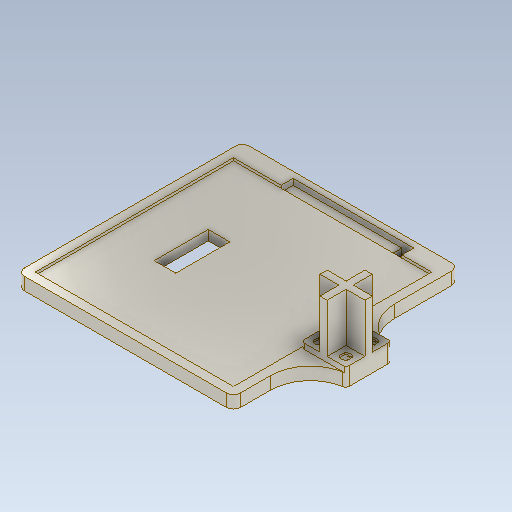
# Autodesk Inventor part: Sun1
Saved by Autodesk Inventor 2021 (Build 250183000, 183)
## iProperties
Created: 2021-04-13
Part Number: Sun1
Material: 티타늄
Document SubType Name: Modeling
Designer: Dongyoon
Density: 4.51 g/cm^3
Appearance: 티타늄
Author: Dongyoon
Autodesk Inventor part; units mm, degrees
ref_plane "YZ Plane" through (0, 0, 0) normal (1, 0, 0) x (0, 1, 0)
sketch "스케치1" plane through (0, 0, 0) normal (0, 1, 0) x (-1, 0, 0)
  line L0 (0, 0) -> (150, 0)
  line L1 (150, 0) -> (150, -140)
  line L2 (150, -140) -> (0, -140)
  line L3 (0, 0) -> (0, -140)
  dimension "d1" = 140
  dimension "d75" = 150
  constraints: 8 end point, 3 perpendicular, 1 horizontal
  measures "d1" distance between parallel lines of L2 L0
  measures "d75" distance between parallel lines of L1 L3
extrude "돌출1" add sketch "스케치1" along normal blind 7
sketch "스케치2" plane through (0, 7, 0) normal (0, 1, 0) x (1, 0, 0)
  line L0 (-145, 130) -> (-25, 130)
  line L1 (-25, 130) -> (-25, 10)
  line L2 (-25, 10) -> (-145, 10)
  line L3 (-145, 10) -> (-145, 130)
  line L4 (-150, 140) -> (-150, 0) projected
  line L5 (0, 140) -> (-150, 140) projected
  point P0 (0, 0)
  dimension "d7" = 120
  dimension "d8" = 120
  dimension "d9" = 5
  dimension "d10" = 10
  constraints: 8 end point, 2 parallel, 1 horizontal, 1 perpendicular
  measures "d7" distance of L1.end L2.end
  measures "d8" distance of L2.end L0.start
  measures "d9" distance between parallel lines of L4 L3
  measures "d10" distance between parallel lines of L5 L0
extrude "돌출2" cut sketch "스케치2" against normal blind 1.5
sketch "스케치3" plane through (0, 7, 0) normal (0, 1, 0) x (1, 0, 0)
  circle A0 centre (-5.25, 77.25) radius 2.55
  line L0 (-7.5, 78.45) -> (-7.5, 76.05)
  line L1 (-3, 76.05) -> (-3, 78.45)
  line L2 (0, 140) -> (-150, 140) projected
  line L3 (-150, 140) -> (-150, 0) projected
  circle A1 centre (-19.75, 62.75) radius 2.55
  line L4 (-22, 63.95) -> (-22, 61.55)
  line L5 (-17.5, 61.55) -> (-17.5, 63.95)
  circle A2 centre (-19.75, 77.25) radius 2.55
  line L6 (-22, 78.45) -> (-22, 76.05)
  line L7 (-17.5, 76.05) -> (-17.5, 78.45)
  circle A3 centre (-5.25, 62.75) radius 2.55
  line L8 (-7.5, 63.95) -> (-7.5, 61.55)
  line L9 (-3, 61.55) -> (-3, 63.95)
  line L10 (-150, 0) -> (0, 0) projected
  line L11 (-25, 130) -> (-25, 10) projected
  line L12 (0, 0) -> (0, 140) projected
  line L13 (-25, 72) -> (0, 72)
  line L14 (-25, 68) -> (0, 68)
  line L15 (-12.5, 72) -> (-12.5, 94.2328)
  line L16 (-12.5, 68) -> (-12.5, 31.3969)
  line L17 (-14.5, 71.4203) -> (-14.5, 94.2328)
  line L18 (-10.5, 71.4203) -> (-10.5, 94.2328)
  line L19 (-14.5, 68) -> (-14.5, 31.3969)
  line L20 (-10.5, 68) -> (-10.5, 31.3969)
  line L21 (-25, 10) -> (-145, 10) projected
  dimension "d13" = 5.1
  dimension "d14" = 4.5
  dimension "d17" = 2.25
  dimension "d18" = 5.1
  dimension "d19" = 4.5
  dimension "d20" = 2.25
  dimension "d21" = 5.1
  dimension "d22" = 4.5
  dimension "d23" = 2.25
  dimension "d24" = 5.1
  dimension "d25" = 4.5
  dimension "d26" = 2.25
  dimension "d99" = 2
  dimension "d100" = 2
  dimension "d101" = 2
  dimension "d102" = 2
  dimension "d107" = 58
  dimension "d108" = 4
  dimension "d112" = 5.25
  dimension "d113" = 5.25
  constraints: 32 end point, 16 point on circle, 8 parallel, 6 vertical, 4 centre point, 2 midpoint
  measures "d13" diameter of A0
  measures "d14" distance between parallel lines of L0 L1
  measures "d17" distance from line of A0.centre L0
  measures "d18" diameter of A1
  measures "d19" distance between parallel lines of L4 L5
  measures "d20" distance from line of A1.centre L4
  measures "d21" diameter of A2
  measures "d22" distance between parallel lines of L6 L7
  measures "d23" distance from line of A2.centre L6
  measures "d24" diameter of A3
  measures "d25" distance between parallel lines of L8 L9
  measures "d26" distance from line of A3.centre L8
  measures "d99" distance between parallel lines of L15 L17
  measures "d100" distance between parallel lines of L15 L18
  measures "d101" distance between parallel lines of L16 L19
  measures "d102" distance between parallel lines of L16 L20
  measures "d107" distance between parallel lines of L21 L14
  measures "d108" distance between parallel lines of L14 L13
  measures "d112" distance from line of L12 A0.centre
  measures "d113" distance from line of L13 A0.centre
extrude "돌출3" cut sketch "스케치3" against normal blind 1 contours L1 A0 L0 | L5 A1 L4 | L7 A2 L6 | L9 A3 L8
sketch "스케치4" plane through (0, 6, 0) normal (0, 1, 0) x (1, 0, 0)
  arc A0 (-17.5, 63.95) -> (-22, 63.95) centre (-19.75, 62.75) ccw projected
  line L0 (-19.3059, 60.239) -> (-20.1941, 65.261) construction
  line L1 (-20.1941, 60.239) -> (-19.3059, 65.261) construction
  arc A1 (-19.3059, 65.261) -> (-20.1941, 65.261) centre (-19.75, 62.75) ccw
  arc A2 (-20.1941, 60.239) -> (-19.3059, 60.239) centre (-19.75, 62.75) ccw
  line L2 (-19.3059, 61.3293) -> (-20.1941, 61.3293)
  line L3 (-20.1941, 64.1707) -> (-19.3059, 64.1707)
  line L4 (-19.3059, 61.3293) -> (-20.1941, 64.1707) construction
  line L5 (-20.1941, 61.3293) -> (-19.3059, 64.1707) construction
  line L6 (-19.3059, 65.261) -> (-19.3059, 64.1707)
  line L7 (-19.3059, 61.3293) -> (-19.3059, 60.239)
  line L8 (-20.1941, 60.239) -> (-20.1941, 61.3293)
  line L9 (-20.1941, 64.1707) -> (-20.1941, 65.261)
  arc A3 (-3, 63.95) -> (-7.5, 63.95) centre (-5.25, 62.75) ccw projected
  arc A4 (-17.5, 78.45) -> (-22, 78.45) centre (-19.75, 77.25) ccw projected
  arc A5 (-3, 78.45) -> (-7.5, 78.45) centre (-5.25, 77.25) ccw projected
  line L10 (-4.8059, 60.239) -> (-5.6941, 65.261) construction
  line L11 (-5.6941, 60.239) -> (-4.8059, 65.261) construction
  arc A6 (-4.8059, 65.261) -> (-5.6941, 65.261) centre (-5.25, 62.75) ccw
  arc A7 (-5.6941, 60.239) -> (-4.8059, 60.239) centre (-5.25, 62.75) ccw
  line L12 (-4.8059, 61.3293) -> (-5.6941, 61.3293)
  line L13 (-5.6941, 64.1707) -> (-4.8059, 64.1707)
  line L14 (-4.8059, 61.3293) -> (-5.6941, 64.1707) construction
  line L15 (-5.6941, 61.3293) -> (-4.8059, 64.1707) construction
  line L16 (-4.8059, 65.261) -> (-4.8059, 64.1707)
  line L17 (-4.8059, 61.3293) -> (-4.8059, 60.239)
  line L18 (-5.6941, 60.239) -> (-5.6941, 61.3293)
  line L19 (-5.6941, 64.1707) -> (-5.6941, 65.261)
  line L20 (-19.3059, 74.739) -> (-20.1941, 79.761) construction
  line L21 (-20.1941, 74.739) -> (-19.3059, 79.761) construction
  arc A8 (-19.3059, 79.761) -> (-20.1941, 79.761) centre (-19.75, 77.25) ccw
  arc A9 (-20.1941, 74.739) -> (-19.3059, 74.739) centre (-19.75, 77.25) ccw
  line L22 (-19.3059, 75.8293) -> (-20.1941, 75.8293)
  line L23 (-20.1941, 78.6707) -> (-19.3059, 78.6707)
  line L24 (-19.3059, 75.8293) -> (-20.1941, 78.6707) construction
  line L25 (-20.1941, 75.8293) -> (-19.3059, 78.6707) construction
  line L26 (-19.3059, 79.761) -> (-19.3059, 78.6707)
  line L27 (-19.3059, 75.8293) -> (-19.3059, 74.739)
  line L28 (-20.1941, 74.739) -> (-20.1941, 75.8293)
  line L29 (-20.1941, 78.6707) -> (-20.1941, 79.761)
  line L30 (-4.8059, 74.739) -> (-5.6941, 79.761) construction
  line L31 (-5.6941, 74.739) -> (-4.8059, 79.761) construction
  arc A10 (-4.8059, 79.761) -> (-5.6941, 79.761) centre (-5.25, 77.25) ccw
  arc A11 (-5.6941, 74.739) -> (-4.8059, 74.739) centre (-5.25, 77.25) ccw
  line L32 (-4.8059, 75.8293) -> (-5.6941, 75.8293)
  line L33 (-5.6941, 78.6707) -> (-4.8059, 78.6707)
  line L34 (-4.8059, 75.8293) -> (-5.6941, 78.6707) construction
  line L35 (-5.6941, 75.8293) -> (-4.8059, 78.6707) construction
  line L36 (-4.8059, 79.761) -> (-4.8059, 78.6707)
  line L37 (-4.8059, 75.8293) -> (-4.8059, 74.739)
  line L38 (-5.6941, 74.739) -> (-5.6941, 75.8293)
  line L39 (-5.6941, 78.6707) -> (-5.6941, 79.761)
  line L40 (-22, 61.55) -> (-22, 63.95) projected
  line L41 (-17.5, 63.95) -> (-17.5, 61.55) projected
  line L42 (-3, 63.95) -> (-3, 61.55) projected
  line L43 (-7.5, 61.55) -> (-7.5, 63.95) projected
  line L44 (-17.5, 78.45) -> (-17.5, 76.05) projected
  line L45 (-3, 78.45) -> (-3, 76.05) projected
  point P0 (0, 0)
  point P1 (-19.3059, 79.761)
  point P2 (-20.1941, 79.761)
  point P3 (-4.8059, 65.261)
  point P4 (-5.6941, 65.261)
  point P5 (-19.3059, 65.261)
  dimension "d43" = 1.8059
  dimension "d44" = 1.8059
  dimension "d45" = 2.8414
  dimension "d46" = 2.55
  dimension "d47" = 2.25
  dimension "d48" = 1.0903
  dimension "d49" = 1.1293
  dimension "d50" = 2.8414
  dimension "d51" = 1.4207
  dimension "d52" = 0.8882
  dimension "d53" = 1.8059
  dimension "d55" = 1.4207
  dimension "d56" = 1.8059
  dimension "d57" = 2.25
  dimension "d58" = 2.55
  dimension "d59" = 1.0903
  dimension "d60" = 1.4207
  dimension "d61" = 2.8414
  dimension "d62" = 0.8882
  dimension "d63" = 0.8882
  dimension "d64" = 1.0903
  dimension "d65" = 1.0903
  dimension "d66" = 1.4207
  dimension "d67" = 1.8059
  dimension "d68" = 1.8059
  dimension "d69" = 1.8059
  dimension "d70" = 2.8414
  dimension "d71" = 1.4207
  dimension "d72" = 1.8059
  dimension "d73" = 0.8882
  dimension "d74" = 0.8882
  constraints: 80 end point, 20 parallel, 18 point on circle, 10 midpoint, 8 centre point, 4 horizontal
  measures "d43" distance between parallel lines of L40 L9
  measures "d44" distance between parallel lines of L41 L6
  measures "d45" distance between parallel lines of L2 L3
  measures "d46" radius of A1
  measures "d47" distance from line of L40 A2.centre
  measures "d48" distance of L1.start L2.end
  measures "d49" distance edge to line of A2 L2
  measures "d50" distance between parallel lines of L12 L13
  measures "d51" distance from line of L13 A6.centre
  measures "d52" distance between parallel lines of L19 L16
  measures "d53" distance between parallel lines of L42 L16
  measures "d55" distance from line of L12 A7.centre
  measures "d56" distance between parallel lines of L43 L18
  measures "d57" distance from line of L43 A6.centre
  measures "d58" radius of A6
  measures "d59" distance from line of L13 L16.start
  measures "d60" distance from line of A3.centre L12
  measures "d61" distance between parallel lines of L22 L23
  measures "d62" distance between parallel lines of L26 L29
  measures "d63" distance between parallel lines of L28 L27
  measures "d64" distance of L26.start L26.end
  measures "d65" distance of L27.start L27.end
  measures "d66" distance from line of A4.centre L22
  measures "d67" distance between parallel lines of L44 L26
  measures "d68" distance between parallel lines of L44 L27
  measures "d69" distance between parallel lines of L45 L36
  measures "d70" distance between parallel lines of L32 L33
  measures "d71" distance from line of L32 A5.centre
  measures "d72" distance between parallel lines of L45 L37
  measures "d73" distance between parallel lines of L38 L37
  measures "d74" distance between parallel lines of L36 L39
extrude "돌출4" cut sketch "스케치4" against normal through all both and the other way through all
sketch "스케치6" plane through (0, 5.5, 0) normal (0, 1, 0) x (1, 0, 0)
  line L0 (-107, 60) -> (-119, 60)
  line L1 (-119, 60) -> (-119, 90)
  line L2 (-119, 90) -> (-107, 90)
  line L3 (-107, 90) -> (-107, 60)
  line L4 (-107, 60) -> (-119, 90) construction
  line L5 (-119, 60) -> (-107, 90) construction
  line L6 (-145, 130) -> (-25, 130) projected
  line L7 (-145, 10) -> (-145, 130) projected
  point P0 (0, 0)
  point P1 (-113, 75)
  dimension "d37" = 12
  dimension "d38" = 30
  dimension "d39" = 55
  dimension "d40" = 32
  constraints: 12 end point, 2 midpoint, 2 parallel, 1 horizontal, 1 perpendicular
  measures "d37" distance of L1.end L2.end
  measures "d38" distance of L2.end L0.start
  measures "d39" distance from line of L6 point (-113, 75)
  measures "d40" distance from line of L7 point (-113, 75)
extrude "돌출5" cut sketch "스케치6" against normal through all
sketch "스케치9" plane through (0, 7, 0) normal (0, 1, 0) x (1, 0, 0)
  line L0 (-25, 130) -> (-25, 10) projected
  line L1 (0, 0) -> (0, 140) projected
  line L2 (-14.5, 82.5) -> (-14.5, 72)
  line L3 (-14.5, 68) -> (-14.5, 57.5)
  line L4 (-10.5, 82.5) -> (-10.5, 72)
  line L5 (-10.5, 68) -> (-10.5, 57.5)
  line L6 (-25, 72) -> (-14.5, 72)
  line L7 (-10.5, 72) -> (0, 72)
  line L8 (-25, 68) -> (-14.5, 68)
  line L9 (-10.5, 68) -> (0, 68)
  line L10 (-25, 10) -> (-145, 10) projected
  line L11 (-145, 130) -> (-25, 130) projected
  line L12 (-14.5, 82.5) -> (-10.5, 82.5)
  line L13 (0, 72) -> (0, 68)
  line L14 (-10.5, 57.5) -> (-14.5, 57.5)
  line L15 (-25, 68) -> (-25, 72)
  line L16 (-25, 130) -> (-25, 10) projected
  point P0 (0, 68)
  point P1 (0, 72)
  dimension "d82" = 4
  dimension "d83" = 4
  dimension "d84" = 10.5
  dimension "d85" = 10.5
  dimension "d86" = 58
  dimension "d87" = 4
  dimension "d88" = 10.5
  dimension "d90" = 10.5
  dimension "d91" = 10.5
  dimension "d92" = 58
  dimension "d93" = 10.5
  dimension "d94" = 10.5
  constraints: 24 end point, 1 collinear, 1 perpendicular
  measures "d82" distance between parallel lines of L8 L6
  measures "d83" distance between parallel lines of L4 L2
  measures "d84" distance between parallel lines of L2 L0
  measures "d85" distance between parallel lines of L3 L0
  measures "d86" distance between parallel lines of L10 L8
  measures "d87" distance between parallel lines of L9 L7
  measures "d88" distance between parallel lines of L1 L5
  measures "d90" distance of L3.start L3.end
  measures "d91" distance of L5.start L5.end
  measures "d92" distance between parallel lines of L10 L9
  measures "d93" distance of L4.start L4.end
  measures "d94" distance of L2.start L2.end
extrude "돌출6" add sketch "스케치9" along normal blind 30
sketch "스케치11" plane through (-14.5, 7, -68) normal (-1, 0, 0) x (0, 0, 1)
  line L0 (0, 0) -> (0, 30) projected
  line L1 (0, 0) -> (10.5, 0)
  line L2 (10.5, 0) -> (10.5, 3)
  line L3 (10.5, 3) -> (0, 3)
  line L4 (0, 3) -> (0, 0)
  point P0 (68, -7)
  point P1 (0, 3)
  dimension "d116" = 10.5
  dimension "d117" = 3
  constraints: 8 end point, 2 parallel, 1 horizontal, 1 perpendicular
  measures "d116" distance of L2.end L3.end
  measures "d117" distance of L1.end L2.end
extrude "돌출7" add sketch "스케치11" along normal up to surface (10.5 mm away)
sketch "스케치12" plane through (-14.5, 10, -57.5) normal (0, 1, 0) x (1, 0, 0)
  arc A0 (-3, 6.45) -> (-7.5, 6.45) centre (-5.25, 5.25) ccw projected
  circle A1 centre (-5.25, 5.25) radius 2.55
  line L0 (-7.5, 4.05) -> (-7.5, 6.45) projected
  line L1 (-7.5, 6.45) -> (-7.5, 4.05)
  line L2 (-3, 6.45) -> (-3, 4.05) projected
  line L3 (-3, 4.05) -> (-3, 6.45)
  point P0 (14.5, -57.5)
  constraints: 4 end point, 1 centre point, 1 coincident, 1 collinear, 1 point on circle
extrude "돌출8" cut sketch "스케치12" against normal blind 3 contours L2 A1 L0 A0
ref_plane "작업 평면1" through (-12.5, 7, -57.5) normal (1, 0, 0) x (0, 0, -1)
mirror "미러1" about plane through (-12.5, 7, -57.5) normal (1, 0, 0) of "돌출8", "돌출7"
ref_plane "작업 평면2" through (-10.5, 37, -70) normal (0, 0, 1) x (1, 0, 0)
mirror "미러2" about plane through (-10.5, 37, -70) normal (0, 0, 1) of "돌출8", "돌출7", "미러1"
sketch "스케치13" plane through (0, 7, 0) normal (0, 1, 0) x (1, 0, 0)
  line L0 (-14.5, 57.5) -> (-25, 57.5) projected
  line L1 (-20, 35.5911) -> (-20, 0)
  line L2 (-150, 0) -> (0, 0) projected
  line L3 (-25, 57.5) -> (-25, 10) projected
  line L4 (-10.5, 57.5) -> (0, 57.5) projected
  arc A0 (0, 57.5) -> (-20, 35.5911) centre (2, 35.5911) ccw
  line L5 (0, 0) -> (0, 57.5) projected
  line L6 (0, 57.5) -> (0, 0)
  line L7 (0, 0) -> (-20, 0)
  dimension "d122" = 5
  dimension "d123" = 22
  constraints: 6 end point, 2 point on circle, 2 vertical, 1 centre point, 1 collinear, 1 point on line, 1 tangent
  measures "d122" distance between parallel lines of L3 L1
  measures "d123" radius of A0
extrude "돌출9" cut sketch "스케치13" against normal through all
mirror "미러3" about plane through (-10.5, 37, -70) normal (0, 0, 1) of "돌출9"
sketch "스케치14" plane through (0, 7, 0) normal (0, 1, 0) x (1, 0, 0)
  line L0 (-145, 130) -> (-25, 130) projected
  line L1 (-108.5, 130) -> (-41.5, 130)
  line L2 (-41.5, 130) -> (-41.5, 136.6)
  line L3 (-41.5, 136.6) -> (-108.5, 136.6)
  line L4 (-108.5, 136.6) -> (-108.5, 130)
  line L5 (-145, 10) -> (-145, 130) projected
  point P0 (0, 0)
  dimension "d126" = 67
  dimension "d127" = 6.6
  dimension "d128" = 36.5
  constraints: 8 end point, 2 parallel, 1 horizontal, 1 perpendicular, 1 point on line
  measures "d126" distance of L2.end L3.end
  measures "d127" distance of L3.end L1.start
  measures "d128" distance between parallel lines of L5 L4
extrude "돌출10" cut sketch "스케치14" against normal blind 3.3
sketch "스케치15" plane through (0, 3.7, 0) normal (0, 1, 0) x (1, 0, 0)
  line L0 (-108.5, 136.6) -> (-41.5, 136.6) projected
  line L1 (-108.5, 130) -> (-41.5, 130) projected
  line L2 (-41.5, 136.6) -> (-48.1, 136.6)
  line L3 (-48.1, 136.6) -> (-48.1, 130)
  line L4 (-48.1, 130) -> (-41.5, 130)
  line L5 (-41.5, 130) -> (-41.5, 136.6)
  point P0 (0, 0)
  dimension "d131" = 6.6
  constraints: 8 end point, 2 parallel, 1 horizontal, 1 perpendicular, 1 point on line
  measures "d131" distance between parallel lines of L5 L3
extrude "돌출11" cut sketch "스케치15" against normal through all
chamfer "모따기1" distance 5 angle 45 1 edges at (-41.5, 0, -133.3)
fillet "모깎기1" radius 2 5 edges at (0, 3.5, -57.5) (0, 3.5, -82.5) (-25, 8.5, -57.5) (-25, 8.5, -82.5) (0, 8.5, -57.5)
sketch "스케치16" plane through (0, 7, 0) normal (0, 1, 0) x (1, 0, 0)
  line L0 (-20, 35.5911) -> (-20, 0) projected
  line L1 (-150, 140) -> (-150, 0) projected
  line L2 (-20, 0) -> (-150, 0)
  line L3 (-150, 0) -> (-150, 5)
  line L4 (-150, 5) -> (-20, 5)
  line L5 (-20, 5) -> (-20, 0)
  line L6 (-25, 10) -> (-145, 10) projected
  point P0 (0, 0)
  dimension "d138" = 5
  constraints: 8 end point, 2 parallel, 1 horizontal, 1 perpendicular, 1 point on line
  measures "d138" distance between parallel lines of L6 L4
extrude "돌출12" cut sketch "스케치16" against normal through all
fillet "모깎기2" radius 4 4 edges at (-150, 3.5, -5) (-20, 3.5, -5) (-20, 3.5, -140) (-150, 3.5, -140)
sketch "스케치17" plane through (0, 6, 0) normal (0, 1, 0) x (1, 0, 0)
  arc A0 (-17.5, 63.95) -> (-22, 63.95) centre (-19.75, 62.75) ccw projected
  circle A1 centre (-19.75, 62.75) radius 2.55
  arc A2 (-22, 61.55) -> (-17.5, 61.55) centre (-19.75, 62.75) ccw projected
  line L0 (-22, 63.95) -> (-22, 61.55)
  line L1 (-17.5, 63.95) -> (-17.5, 61.55)
  line L2 (-20.1941, 61.3293) -> (-20.1941, 60.239) projected
  line L3 (-19.3059, 61.3293) -> (-20.1941, 61.3293) projected
  line L4 (-20.1941, 60.239) -> (-20.1941, 61.3293)
  line L5 (-19.3059, 60.239) -> (-19.3059, 61.3293) projected
  line L6 (-20.1941, 61.3293) -> (-19.3059, 61.3293)
  line L7 (-19.3059, 61.3293) -> (-19.3059, 60.239)
  line L8 (-20.1941, 65.261) -> (-20.1941, 64.1707) projected
  line L9 (-20.1941, 64.1707) -> (-19.3059, 64.1707) projected
  line L10 (-20.1941, 65.261) -> (-20.1941, 64.1707)
  line L11 (-20.1941, 64.1707) -> (-19.3059, 64.1707)
  line L12 (-19.3059, 64.1707) -> (-19.3059, 65.261)
  line L13 (-7.5, 61.55) -> (-7.5, 63.95) projected
  line L14 (-7.5, 63.95) -> (-7.5, 61.55)
  line L15 (-7.5, 76.05) -> (-7.5, 78.45) projected
  arc A3 (-7.5, 76.05) -> (-3, 76.05) centre (-5.25, 77.25) ccw projected
  line L16 (-7.5, 78.45) -> (-7.5, 76.05)
  arc A4 (-17.5, 78.45) -> (-22, 78.45) centre (-19.75, 77.25) ccw projected
  arc A5 (-22, 76.05) -> (-17.5, 76.05) centre (-19.75, 77.25) ccw projected
  line L17 (-22, 78.45) -> (-22, 76.05)
  circle A6 centre (-5.25, 62.75) radius 2.55
  line L18 (-7.5, 63.95) -> (-7.5, 61.55)
  line L19 (-3, 63.95) -> (-3, 61.55)
  line L20 (-5.6941, 60.239) -> (-5.6941, 61.3293)
  line L21 (-5.6941, 61.3293) -> (-4.8059, 61.3293)
  line L22 (-4.8059, 61.3293) -> (-4.8059, 60.239)
  line L23 (-5.6941, 65.261) -> (-5.6941, 64.1707)
  line L24 (-5.6941, 64.1707) -> (-4.8059, 64.1707)
  line L25 (-4.8059, 64.1707) -> (-4.8059, 65.261)
  circle A7 centre (-5.25, 77.25) radius 2.55
  line L26 (-7.5, 78.45) -> (-7.5, 76.05)
  line L27 (-3, 78.45) -> (-3, 76.05)
  line L28 (-5.6941, 74.739) -> (-5.6941, 75.8293)
  line L29 (-5.6941, 75.8293) -> (-4.8059, 75.8293)
  line L30 (-4.8059, 75.8293) -> (-4.8059, 74.739)
  line L31 (-5.6941, 79.761) -> (-5.6941, 78.6707)
  line L32 (-5.6941, 78.6707) -> (-4.8059, 78.6707)
  line L33 (-4.8059, 78.6707) -> (-4.8059, 79.761)
  circle A8 centre (-19.75, 77.25) radius 2.55
  line L34 (-22, 78.45) -> (-22, 76.05)
  line L35 (-17.5, 78.45) -> (-17.5, 76.05)
  line L36 (-20.1941, 74.739) -> (-20.1941, 75.8293)
  line L37 (-20.1941, 75.8293) -> (-19.3059, 75.8293)
  line L38 (-19.3059, 75.8293) -> (-19.3059, 74.739)
  line L39 (-20.1941, 79.761) -> (-20.1941, 78.6707)
  line L40 (-20.1941, 78.6707) -> (-19.3059, 78.6707)
  line L41 (-19.3059, 78.6707) -> (-19.3059, 79.761)
  point P0 (0, 0)
  point P1 (-3, 76.05)
  constraints: 70 end point, 15 perpendicular, 11 vertical, 9 point on circle, 4 centre point, 1 coincident
extrude "돌출13" add sketch "스케치17" along normal blind 3 contours L1 A1 L5 L3 L2 L0 A0 L8 L9 L12 | L13 A6 L23 L24 L25 L19 L22 L21 L20 | L15 A7 L31 L32 L33 L27 A3 L30 L29 L28 | L35 A5 L38 L37 L36 L17 A4 L39 L40 L41
sketch "스케치19" plane through (0, 5.5, 0) normal (0, 1, 0) x (1, 0, 0)
  line L0 (-41.5, 130) -> (-25, 130) projected
  line L1 (-25, 130) -> (-135, 130)
  line L2 (-135, 130) -> (-135, 20)
  line L3 (-135, 20) -> (-25, 20)
  line L4 (-25, 20) -> (-25, 130)
  line L5 (-145, 10) -> (-145, 130) projected
  line L6 (-135, 130) -> (-145, 130)
  line L7 (-25, 10) -> (-145, 10) projected
  line L8 (-145, 130) -> (-145, 10)
  line L9 (-145, 10) -> (-25, 10)
  line L10 (-25, 10) -> (-25, 20)
  line L11 (-20, 35.5911) -> (-20, 9) projected
  point P0 (0, 0)
  dimension "d144" = 110
  dimension "d145" = 110
  constraints: 16 end point, 4 perpendicular, 3 parallel, 1 horizontal
  measures "d144" distance of L2.end L3.end
  measures "d145" distance of L1.end L2.end
extrude "돌출14" add sketch "스케치19" along normal up to surface (1.5 mm away) contours L2 L3 L10 L7 L5 L6
sketch "스케치20" plane through (0, 5.5, 0) normal (0, 1, 0) x (1, 0, 0)
  line L0 (-107, 90) -> (-119, 90) projected
  line L1 (-109, 90) -> (-97, 90)
  line L2 (-97, 90) -> (-97, 60)
  line L3 (-97, 60) -> (-109, 60)
  line L4 (-109, 60) -> (-109, 90)
  line L5 (-135, 130) -> (-135, 20) projected
  point P0 (0, 0)
  dimension "d151" = 12
  dimension "d152" = 30
  dimension "d153" = 26
  constraints: 8 end point, 2 parallel, 1 horizontal, 1 perpendicular, 1 point on line
  measures "d151" distance of L1.start L1.end
  measures "d152" distance of L1.end L2.end
  measures "d153" distance between parallel lines of L5 L4
sketch "스케치21" plane through (0, 0, 0) normal (0, -1, 0) x (1, 0, 0)
  line L0 (-107, -60) -> (-107, -90) projected
  line L1 (-107, -90) -> (-119, -90)
  line L2 (-119, -90) -> (-119, -60)
  line L3 (-119, -60) -> (-107, -60)
  line L4 (-107, -60) -> (-107, -90)
  point P0 (0, 0)
  constraints: 8 end point, 2 parallel, 1 horizontal, 1 perpendicular
extrude "돌출15" add sketch "스케치21" against normal up to surface (5.5 mm away)
extrude "돌출16" cut sketch "스케치20" against normal blind 10
sketch "스케치22" plane through (0, 7, 0) normal (0, 1, 0) x (1, 0, 0)
  line L0 (-24, 140) -> (-146, 140) projected
  line L1 (-140, 140) -> (-150, 140)
  line L2 (-150, 140) -> (-150, 5)
  line L3 (-150, 5) -> (-140, 5)
  line L4 (-140, 15) -> (-140, 140)
  line L5 (-20, 9) -> (-20, 35.5911) projected
  line L6 (-150, 5) -> (-20, 5)
  line L7 (-20, 5) -> (-20, 15)
  line L8 (-20, 15) -> (-140, 15)
  line L9 (-150, 15) -> (-150, 5)
  point P0 (0, 0)
  dimension "d156" = 10
  dimension "d157" = 10
  constraints: 16 end point, 4 parallel, 2 horizontal, 2 perpendicular, 2 point on line
  measures "d156" distance between parallel lines of L6 L8
  measures "d157" distance between parallel lines of L4 L2
extrude "돌출17" cut sketch "스케치22" against normal blind 10
fillet "모깎기3" radius 4 3 edges at (-20, 3.5, -15) (-140, 3.5, -15) (-140, 3.5, -140)
